Autodesk Inventor part; units mm, degrees
(part 16 of 18)
  line L724 (-5.504, -21.7643) -> (-5.5203, -21.8411)
  arc A19 (7.2375, -23.8979) -> (7.3559, -23.8917) centre (7.2339, -22.6979) ccw
  line L725 (7.7084, -21.9119) -> (7.7586, -22.8684)
  line L726 (6.7189, -22.7122) -> (6.7222, -22.7735)
  arc A20 (9.7799, -23.0242) -> (10.2699, -22.9899) centre (9.9431, -21.8353) ccw
  line L727 (11.0395, -10.3654) -> (11.03, -10.5528)
  line L728 (10.9782, -11.575) -> (10.9727, -11.6853)
  line L729 (10.6615, -17.8311) -> (10.5427, -20.1764)
  line L730 (10.4882, -21.2523) -> (10.4537, -21.9338)
  line L731 (-9.1815, -10.4211) -> (-9.1812, -10.4622)
  line L732 (-9.1335, -17.7807) -> (-9.1304, -18.2698)
  line L733 (8.997, -17.6632) -> (9.1469, -19.1987)
  line L734 (-8.9887, -17.6618) -> (-9.1388, -19.1973)
  line L735 (9.1909, -10.4225) -> (9.1906, -10.4636)
  line L736 (9.1419, -17.7714) -> (9.1385, -18.2712)
  ellipse E590 centre (-10.1862, -4.6596) end of major axis (-11.8856, -4.7023) minor radius 0.2846 (-11.3721, -4.4846) -> (-11.8856, -4.7023) ccw
  line L737 (-11.8818, -4.8559) -> (-11.8856, -4.7023)
  ellipse E591 centre (10.1964, -4.6611) end of major axis (11.8959, -4.7041) minor radius 0.2846 (11.8959, -4.7041) -> (11.3824, -4.4863) ccw
  line L738 (11.892, -4.8577) -> (11.8959, -4.7041)
  ellipse E592 centre (-10.7093, -6.5045) end of major axis (-12.4071, -6.5902) minor radius 0.3038 (-11.6572, -6.2984) -> (-12.4071, -6.5902) ccw
  line L739 (-12.3999, -6.7335) -> (-12.4071, -6.5902)
  ellipse E593 centre (10.7192, -6.5061) end of major axis (12.4171, -6.5921) minor radius 0.3038 (12.4171, -6.5921) -> (11.6673, -6.3002) ccw
  line L740 (12.4098, -6.7354) -> (12.4171, -6.5921)
  ellipse E594 centre (7.1057, -3.5892) end of major axis (8.7977, -3.4241) minor radius 0.0977 (8.7977, -3.4241) -> (8.2803, -3.4043) ccw
  line L741 (8.8221, -3.6736) -> (8.7977, -3.4241)
  ellipse E595 centre (-7.0953, -3.5881) end of major axis (-8.7872, -3.4227) minor radius 0.0977 (-8.2699, -3.403) -> (-8.7872, -3.4227) ccw
  line L742 (-8.8116, -3.6723) -> (-8.7872, -3.4227)
  ellipse E596 centre (-10.1094, -7.7149) end of major axis (-8.6099, -7.6772) minor radius 0.2511 (-9.2363, -7.4893) -> (-9.8598, -7.4611) ccw
  ellipse E597 centre (-10.1094, -7.7149) end of major axis (-8.21, -7.6671) minor radius 0.3181 (-9.2281, -7.4115) -> (-11.1736, -7.4773) ccw
  ellipse E598 centre (-10.1787, -4.9552) end of major axis (-12.0781, -5.003) minor radius 0.3181 (-10.8806, -4.6767) -> (-12.0781, -5.003) ccw
  line L743 (-12.0435, -6.3816) -> (-12.0781, -5.003)
  ellipse E599 centre (7.4558, -8.6381) end of major axis (9.3455, -8.4403) minor radius 0.0812 (9.1873, -8.4899) -> (9.1288, -8.4254) ccw
  ellipse E600 centre (7.1646, -5.8558) end of major axis (9.0543, -5.6581) minor radius 0.0812 (8.9436, -5.6425) -> (8.5431, -5.656) ccw
  line L744 (9.3455, -8.4403) -> (9.1404, -6.481)
  ellipse E601 centre (-7.4461, -8.6369) end of major axis (-9.3358, -8.4389) minor radius 0.0812 (-9.1191, -8.424) -> (-9.1776, -8.4885) ccw
  ellipse E602 centre (-7.1546, -5.8547) end of major axis (-9.0442, -5.6567) minor radius 0.0812 (-8.533, -5.6547) -> (-8.9335, -5.6411) ccw
  line L745 (-9.3358, -8.4389) -> (-9.1305, -6.4796)
  ellipse E603 centre (10.1192, -7.7164) end of major axis (11.6187, -7.7543) minor radius 0.2511 (9.8697, -7.4626) -> (9.2461, -7.4907) ccw
  ellipse E604 centre (10.1192, -7.7164) end of major axis (12.0186, -7.7644) minor radius 0.3181 (11.1834, -7.479) -> (9.238, -7.4129) ccw
  ellipse E605 centre (10.1889, -4.9568) end of major axis (12.0883, -5.0048) minor radius 0.3181 (12.0883, -5.0048) -> (10.8909, -4.6784) ccw
  line L746 (12.0535, -6.3834) -> (12.0883, -5.0048)
  ellipse E606 centre (-10.5555, -9.5507) end of major axis (-12.0536, -9.6263) minor radius 0.2681 (-9.2747, -9.3489) -> (-11.7458, -9.7719) ccw
  ellipse E607 centre (-10.5555, -9.5507) end of major axis (-12.4531, -9.6465) minor radius 0.3396 (-9.2623, -9.2387) -> (-11.7407, -9.8742) ccw
  ellipse E608 centre (-10.6944, -6.7993) end of major axis (-12.592, -6.8951) minor radius 0.3396 (-11.2097, -6.4972) -> (-12.592, -6.8951) ccw
  line L747 (-12.4531, -9.6465) -> (-12.592, -6.8951)
  ellipse E609 centre (7.5123, -10.5929) end of major axis (9.4003, -10.3801) minor radius 0.0405 (9.1011, -10.4359) -> (9.096, -10.3923) ccw
  ellipse E610 centre (7.1988, -7.8111) end of major axis (9.0868, -7.5984) minor radius 0.0405 (9.0374, -7.5948) -> (8.7713, -7.6115) ccw
  line L748 (9.4003, -10.3801) -> (9.1815, -8.4386)
  ellipse E611 centre (-7.5029, -10.5918) end of major axis (-9.3909, -10.3787) minor radius 0.0405 (-9.0866, -10.3909) -> (-9.0917, -10.4345) ccw
  ellipse E612 centre (-7.189, -7.8101) end of major axis (-9.077, -7.597) minor radius 0.0405 (-8.7615, -7.6101) -> (-9.0276, -7.5934) ccw
  line L749 (-9.3909, -10.3787) -> (-9.1718, -8.4372)
  ellipse E613 centre (10.565, -9.5523) end of major axis (12.0631, -9.6282) minor radius 0.2681 (11.7553, -9.7736) -> (9.2843, -9.3503) ccw
  ellipse E614 centre (10.565, -9.5523) end of major axis (12.4626, -9.6484) minor radius 0.3396 (11.7501, -9.8759) -> (9.2718, -9.2401) ccw
  ellipse E615 centre (10.7043, -6.8009) end of major axis (12.6019, -6.897) minor radius 0.3396 (12.6019, -6.897) -> (11.2197, -6.499) ccw
  line L750 (12.4626, -9.6484) -> (12.6019, -6.897)
  ellipse E616 centre (-9.7263, -5.8407) end of major axis (-8.2264, -5.8309) minor radius 0.2359 (-9.2027, -5.6163) -> (-9.2198, -5.6155) ccw
  ellipse E617 centre (-9.7263, -5.8407) end of major axis (-7.8264, -5.8283) minor radius 0.2988 (-9.1962, -5.5504) -> (-10.8665, -5.6089) ccw
  ellipse E618 centre (-9.7443, -3.0756) end of major axis (-11.6443, -3.088) minor radius 0.2988 (-11.5643, -3.0014) -> (-11.6443, -3.088) ccw
  line L751 (-11.6348, -4.5461) -> (-11.6443, -3.088)
  ellipse E619 centre (7.4064, -6.6695) end of major axis (9.2974, -6.4849) minor radius 0.1092 (9.1469, -6.543) -> (9.0264, -6.4553) ccw
  ellipse E620 centre (7.1348, -3.8873) end of major axis (9.0258, -3.7027) minor radius 0.1092 (9.0258, -3.7027) -> (8.3133, -3.6868) ccw
  line L752 (9.2974, -6.4849) -> (9.0258, -3.7027)
  ellipse E621 centre (-7.3965, -6.6683) end of major axis (-9.2874, -6.4835) minor radius 0.1092 (-9.0164, -6.4539) -> (-9.137, -6.5416) ccw
  ellipse E622 centre (-7.1245, -3.8862) end of major axis (-9.0154, -3.7014) minor radius 0.1092 (-8.3029, -3.6856) -> (-9.0154, -3.7014) ccw
  line L753 (-9.2874, -6.4835) -> (-9.0154, -3.7014)
  ellipse E623 centre (9.7364, -5.8422) end of major axis (11.2364, -5.8522) minor radius 0.2359 (9.23, -5.6169) -> (9.2128, -5.6177) ccw
  ellipse E624 centre (9.7364, -5.8422) end of major axis (11.6364, -5.8548) minor radius 0.2988 (10.8767, -5.6106) -> (9.2063, -5.5518) ccw
  ellipse E625 centre (9.7548, -3.0771) end of major axis (11.6548, -3.0897) minor radius 0.2988 (11.6548, -3.0897) -> (11.5748, -3.0032) ccw
  line L754 (11.6451, -4.5478) -> (11.6548, -3.0897)
  line L755 (-8.7402, -12.0526) -> (-8.7237, -12.1531)
  line L756 (-8.7073, -12.253) -> (-7.5133, -19.5411)
  line L757 (-3.535, -19.9576) -> (-2.6762, -17.7502)
  line L758 (-3.5351, -19.9577) -> (-3.535, -19.9576)
  line L759 (-8.1616, -6.5272) -> (-8.5418, -10.158)
  line L760 (-8.7397, -12.0478) -> (-8.7402, -12.0526)
  line L761 (-8.1617, -6.5272) -> (-8.2376, -7.2524)
  line L762 (-3.607, -19.9502) -> (-3.5351, -19.9577)
  line L763 (-7.5133, -19.5411) -> (-7.0907, -19.5854)
  line L764 (-5.4323, -19.759) -> (-3.535, -19.9576)
  ellipse E626 centre (-8.1618, -6.5272) end of major axis (-8.2147, -7.0324) minor radius 0.0001 (-8.1617, -6.5272) -> (-8.1373, -6.2939) ccw
  ellipse E627 centre (-8.1618, -6.5272) end of major axis (-8.2676, -7.5377) minor radius 0.0002 (-8.1616, -6.5272) -> (-8.1128, -6.0606) ccw
  ellipse E628 centre (-7.4804, -0.0138) end of major axis (-7.3746, 0.9967) minor radius 0.0002 (-7.4314, 0.4529) -> (-7.3746, 0.9967) ccw
  ellipse E629 centre (-7.4804, -0.0138) end of major axis (-7.4275, 0.4915) minor radius 0.0001 (-7.4559, 0.2195) -> (-7.4275, 0.4915) ccw
  line L765 (-7.3746, 0.9967) -> (-7.0642, 0.9642)
  line L766 (-8.1373, -6.2939) -> (-7.4559, 0.2195)
  line L767 (-8.1128, -6.0606) -> (-7.4314, 0.4529)
  line L768 (-7.3747, 0.9966) -> (-8.3698, 1.1006)
  line L769 (-8.4227, 0.5954) -> (-8.3698, 1.1006)
  line L770 (-8.4227, 0.5954) -> (-7.4276, 0.4914)
  line L771 (-7.3747, 0.9966) -> (-7.4276, 0.4914)
  line L772 (-8.3698, 1.1006) -> (-8.3699, 1.1006)
  line L773 (-7.4276, 0.4914) -> (-7.4275, 0.4915)
  line L774 (-7.3746, 0.9967) -> (-7.3747, 0.9966)
  line L775 (-3.9949, -5.5989) -> (-3.995, -6.2751)
  line L776 (4.0051, -5.5995) -> (4.005, -6.2757)
  line L777 (-3.9949, -5.5989) -> (-3.9949, -5.1443)
  line L778 (4.0051, -5.5995) -> (4.0051, -5.1449)
  line L779 (-3.9949, -5.1443) -> (-3.9949, -4.6721)
  line L780 (4.0051, -4.6727) -> (4.0051, -5.1449)
  line L781 (4.3271, 1.2542) -> (4.0056, 1.36)
  line L782 (4.0055, 0.8547) -> (4.2649, 0.7694)
  line L783 (-3.9944, 1.3606) -> (-4.3159, 1.2549)
  line L784 (-4.2538, 0.7701) -> (-3.9945, 0.8553)
  line L785 (3.543, -19.9582) -> (3.5431, -19.9582)
  line L786 (2.6845, -17.7506) -> (3.543, -19.9582)
  line L787 (7.5213, -19.5423) -> (8.7164, -12.2543)
  line L788 (8.7328, -12.1544) -> (8.7493, -12.054)
  line L789 (8.2475, -7.2537) -> (8.1717, -6.5284)
  line L790 (8.1716, -6.5284) -> (8.5512, -10.1593)
  line L791 (8.7488, -12.0492) -> (8.7493, -12.054)
  line L792 (3.5431, -19.9582) -> (3.6149, -19.9507)
  line L793 (3.543, -19.9582) -> (5.4402, -19.7598)
  line L794 (7.0987, -19.5864) -> (7.5213, -19.5423)
  ellipse E630 centre (8.1718, -6.5285) end of major axis (8.119, -6.0232) minor radius 0.0001 (8.1473, -6.2951) -> (8.1717, -6.5284) ccw
  ellipse E631 centre (8.1718, -6.5285) end of major axis (8.2774, -7.5389) minor radius 0.0002 (8.1228, -6.0618) -> (8.1716, -6.5284) ccw
  ellipse E632 centre (7.4913, -0.0149) end of major axis (7.3857, 0.9956) minor radius 0.0002 (7.3857, 0.9956) -> (7.4424, 0.4517) ccw
  ellipse E633 centre (7.4913, -0.0149) end of major axis (7.4385, 0.4903) minor radius 0.0001 (7.4385, 0.4903) -> (7.4669, 0.2184) ccw
  line L795 (7.0753, 0.9631) -> (7.3857, 0.9956)
  line L796 (8.1473, -6.2951) -> (7.4669, 0.2184)
  line L797 (7.4424, 0.4517) -> (8.1228, -6.0618)
  line L798 (8.3809, 1.0993) -> (7.3858, 0.9955)
  line L799 (7.4387, 0.4903) -> (7.3858, 0.9955)
  line L800 (7.4387, 0.4903) -> (8.4338, 0.5941)
  line L801 (8.4338, 0.5941) -> (8.3809, 1.0993)
  line L802 (8.381, 1.0993) -> (8.3809, 1.0993)
  line L803 (7.3858, 0.9955) -> (7.3857, 0.9956)
  line L804 (7.4385, 0.4903) -> (7.4387, 0.4903)
  line L805 (-2.9778, -18.5255) -> (-1.9962, -22.1194)
  line L806 (2.0038, -22.1197) -> (2.986, -18.5259)
  line L807 (-1.9962, -22.1194) -> (2.0038, -22.1197)
  line L808 (-2.3716, -21.7977) -> (-1.9963, -23.1626)
  line L809 (2.0037, -23.1629) -> (2.3767, -21.8074)
  line L810 (-1.9963, -23.1626) -> (2.0037, -23.1629)
  line L811 (-8.3636, -21.43) -> (-9.5, -13.9273)
  line L812 (-8.3635, -21.43) -> (-8.3636, -21.43)
  line L813 (-9.5, -13.9273) -> (-8.3635, -21.43)
  line L814 (-9.5, -13.9273) -> (-9.5, -13.9273)
  line L815 (-4.3906, -21.8945) -> (-3.607, -19.9501)
  line L816 (-4.3906, -21.8945) -> (-4.3906, -21.8945)
  line L817 (-8.8548, -8.4092) -> (-9.5, -13.9273)
  line L818 (-8.8549, -8.4092) -> (-9.5, -13.9273)
  line L819 (-8.3636, -21.43) -> (-4.3906, -21.8945)
  line L820 (-8.3635, -21.43) -> (-4.3906, -21.8945)
  ellipse E634 centre (-8.8549, -8.4092) end of major axis (-8.9139, -8.9138) minor radius 0 (-8.8549, -8.4092) -> (-8.8277, -8.1762) ccw
  ellipse E635 centre (-8.8549, -8.4092) end of major axis (-8.9729, -9.4183) minor radius 0.0001 (-8.8548, -8.4092) -> (-8.8004, -7.9432) ccw
  ellipse E636 centre (-8.0948, -1.9044) end of major axis (-7.9768, -0.8953) minor radius 0.0001 (-8.0402, -1.4384) -> (-7.9768, -0.8953) ccw
  ellipse E637 centre (-8.0948, -1.9044) end of major axis (-8.0358, -1.3999) minor radius 0 (-8.0675, -1.6714) -> (-8.0358, -1.3999) ccw
  line L821 (-7.9768, -0.8953) -> (-7.5774, -0.942)
  line L822 (-8.8277, -8.1762) -> (-8.0675, -1.6714)
  line L823 (-8.8004, -7.9432) -> (-8.0402, -1.4384)
  line L824 (-7.9769, -0.8953) -> (-8.9705, -0.7793)
  line L825 (-9.0294, -1.2839) -> (-8.9705, -0.7793)
  line L826 (-9.0294, -1.2839) -> (-8.0359, -1.3999)
  line L827 (-7.9769, -0.8953) -> (-8.0359, -1.3999)
  line L828 (-8.9705, -0.7793) -> (-8.9705, -0.7794)
  line L829 (-8.0359, -1.3999) -> (-8.0358, -1.3999)
  line L830 (-7.9768, -0.8953) -> (-7.9769, -0.8953)
  line L831 (-1.9961, -20.2236) -> (-3.9955, -12.9528)
  line L832 (-1.996, -20.1647) -> (-1.9961, -20.2236)
  line L833 (-3.9955, -12.8939) -> (-1.996, -20.1647)
  line L834 (-3.9955, -12.9528) -> (-3.9955, -12.8939)
  line L835 (4.0045, -12.9534) -> (2.0039, -20.2239)
  line L836 (4.0045, -12.8945) -> (4.0045, -12.9534)
  line L837 (2.004, -20.165) -> (4.0045, -12.8945)
  line L838 (2.0039, -20.2239) -> (2.004, -20.165)
  line L839 (-3.9951, -7.3757) -> (-3.9955, -12.8939)
  line L840 (4.0049, -7.3763) -> (4.0045, -12.8945)
  line L841 (-1.9961, -20.2236) -> (2.0039, -20.2239)
  line L842 (-1.996, -20.1647) -> (2.004, -20.165)
  line L843 (-3.9951, -7.3757) -> (-3.995, -6.923)
  line L844 (4.0049, -7.3763) -> (4.005, -6.9236)
  line L845 (-3.995, -6.923) -> (-3.995, -6.2751)
  line L846 (4.005, -6.2757) -> (4.005, -6.9236)
  line L847 (4.218, -0.5689) -> (4.0054, -0.491)
  line L848 (4.0054, -0.9955) -> (4.158, -1.0515)
  line L849 (-3.9946, -0.4904) -> (-4.2071, -0.5682)
  line L850 (-4.1472, -1.0508) -> (-3.9946, -0.9949)
  line L851 (4.3982, -21.8952) -> (4.3983, -21.8952)
  line L852 (3.6149, -19.9507) -> (4.3982, -21.8952)
  line L853 (9.5089, -13.9287) -> (8.3713, -21.4313)
  line L854 (9.5088, -13.9287) -> (9.5089, -13.9287)
  line L855 (8.3712, -21.4313) -> (9.5088, -13.9287)
  line L856 (8.3713, -21.4313) -> (8.3712, -21.4313)
  line L857 (9.5089, -13.9287) -> (8.8646, -8.4105)
  line L858 (8.8645, -8.4105) -> (9.5088, -13.9287)
  line L859 (4.3983, -21.8952) -> (8.3713, -21.4313)
  line L860 (4.3982, -21.8952) -> (8.3712, -21.4313)
  ellipse E638 centre (8.8646, -8.4105) end of major axis (8.8057, -7.906) minor radius 0 (8.8374, -8.1775) -> (8.8646, -8.4105) ccw
  ellipse E639 centre (8.8646, -8.4105) end of major axis (8.9825, -9.4197) minor radius 0.0001 (8.8101, -7.9445) -> (8.8645, -8.4105) ccw
  ellipse E640 centre (8.1055, -1.9056) end of major axis (7.9876, -0.8965) minor radius 0.0001 (7.9876, -0.8965) -> (8.051, -1.4396) ccw
  ellipse E641 centre (8.1055, -1.9056) end of major axis (8.0465, -1.4011) minor radius 0 (8.0465, -1.4011) -> (8.0782, -1.6726) ccw
  line L861 (7.5882, -0.9431) -> (7.9876, -0.8965)
  line L862 (8.8374, -8.1775) -> (8.0782, -1.6726)
  line L863 (8.051, -1.4396) -> (8.8101, -7.9445)
  line L864 (8.9813, -0.7807) -> (7.9877, -0.8965)
  line L865 (8.0466, -1.4011) -> (7.9877, -0.8965)
  line L866 (8.0466, -1.4011) -> (9.0402, -1.2853)
  line L867 (9.0402, -1.2853) -> (8.9813, -0.7807)
  line L868 (8.9814, -0.7807) -> (8.9813, -0.7807)
  line L869 (7.9877, -0.8965) -> (7.9876, -0.8965)
  line L870 (8.0465, -1.4011) -> (8.0466, -1.4011)
  line L871 (-7.5936, -4.6189) -> (-7.7747, -6.5283)
  line L872 (-7.5936, -4.6189) -> (-7.6627, -5.3469)
  ellipse E642 centre (-7.5936, -4.6189) end of major axis (-7.6416, -5.1246) minor radius 0 (-7.5936, -4.6189) -> (-7.5714, -4.3854) ccw
  ellipse E643 centre (-7.5936, -4.6189) end of major axis (-7.6896, -5.6304) minor radius 0.0001 (-7.5936, -4.6189) -> (-7.5493, -4.1518) ccw
  ellipse E644 centre (-6.9754, 1.901) end of major axis (-6.8794, 2.9125) minor radius 0.0001 (-6.931, 2.3681) -> (-6.8794, 2.9125) ccw
  ellipse E645 centre (-6.9754, 1.901) end of major axis (-6.9274, 2.4068) minor radius 0 (-6.9532, 2.1346) -> (-6.9274, 2.4068) ccw
  line L873 (-6.8794, 2.9125) -> (-4.5993, 2.6962)
  line L874 (-7.5714, -4.3854) -> (-6.9532, 2.1346)
  line L875 (-7.5493, -4.1518) -> (-6.931, 2.3681)
  line L876 (-6.8795, 2.9125) -> (-7.8752, 3.0069)
  line L877 (-7.9232, 2.5012) -> (-7.8752, 3.0069)
  line L878 (-7.9232, 2.5012) -> (-6.9275, 2.4068)
  line L879 (-6.8795, 2.9125) -> (-6.9275, 2.4068)
  line L880 (-7.8752, 3.0069) -> (-7.8754, 3.0069)
  line L881 (-6.9275, 2.4068) -> (-6.9274, 2.4068)
  line L882 (-6.8794, 2.9125) -> (-6.8795, 2.9125)
  line L883 (-3.9948, -3.7775) -> (-3.9949, -4.6721)
  line L884 (4.0052, -3.7782) -> (4.0051, -4.6727)
  line L885 (-3.9948, -3.7775) -> (-3.9948, -3.3213)
  line L886 (4.0052, -3.7782) -> (4.0052, -3.3219)
  line L887 (4.0057, 2.8765) -> (4.0057, 3.3404)
  line L888 (-3.9943, 3.3411) -> (-3.9943, 2.8771)
  line L889 (-3.9943, 3.3411) -> (4.0057, 3.3404)
  line L890 (-3.9948, -3.3213) -> (-3.9943, 2.8771)
  line L891 (4.0057, 2.8765) -> (4.0052, -3.3219)
  line L892 (5.0057, 2.9434) -> (4.0057, 3.2416)
  line L893 (4.0057, 2.7359) -> (4.4825, 2.5937)
  line L894 (5.0057, 2.7329) -> (5.0057, 2.9434)
  line L895 (-3.9943, 3.2422) -> (-4.9943, 2.9442)
  line L896 (-4.9943, 2.7337) -> (-4.9943, 2.9442)
  line L897 (-4.4711, 2.5944) -> (-3.9943, 2.7365)
  line L898 (7.6728, -5.3481) -> (7.6039, -4.62)
  line L899 (7.6038, -4.62) -> (7.7847, -6.5295)
  ellipse E646 centre (7.6039, -4.62) end of major axis (7.556, -4.1143) minor radius 0 (7.5817, -4.3865) -> (7.6039, -4.62) ccw
  ellipse E647 centre (7.6039, -4.62) end of major axis (7.6997, -5.6315) minor radius 0.0001 (7.5596, -4.153) -> (7.6038, -4.62) ccw
  ellipse E648 centre (6.9866, 1.9) end of major axis (6.8908, 2.9115) minor radius 0.0001 (6.8908, 2.9115) -> (6.9423, 2.367) ccw
  ellipse E649 centre (6.9866, 1.9) end of major axis (6.9387, 2.4057) minor radius 0 (6.9387, 2.4057) -> (6.9645, 2.1335) ccw
  line L900 (4.6106, 2.6955) -> (6.8908, 2.9115)
  line L901 (7.5817, -4.3865) -> (6.9645, 2.1335)
  line L902 (6.9423, 2.367) -> (7.5596, -4.153)
  line L903 (7.8867, 3.0057) -> (6.8909, 2.9115)
  line L904 (6.9388, 2.4057) -> (6.8909, 2.9115)
  line L905 (6.9388, 2.4057) -> (7.9346, 2.5)
  line L906 (7.9346, 2.5) -> (7.8867, 3.0057)
  line L907 (7.8868, 3.0057) -> (7.8867, 3.0057)
  line L908 (6.8909, 2.9115) -> (6.8908, 2.9115)
  line L909 (6.9387, 2.4057) -> (6.9388, 2.4057)
  line L910 (-7.7768, -8.2773) -> (-7.756, -8.0785)
  line L911 (-7.7557, -8.0785) -> (-7.7766, -8.2774)
  line L912 (-7.756, -8.0785) -> (-7.7557, -8.0785)
  line L913 (-8.0252, -8.2513) -> (-8.0254, -8.2514)
  line L914 (-7.7766, -8.2774) -> (-8.0252, -8.2513)
  line L915 (-6.782, -8.3815) -> (-6.7612, -8.1826)
  line L916 (-6.5334, -8.4075) -> (-6.782, -8.3815)
  line L917 (-6.7315, -10.2973) -> (-6.9799, -10.2713)
  line L918 (-6.7312, -10.2972) -> (-6.7315, -10.2973)
  line L919 (-7.0007, -10.4701) -> (-6.9799, -10.2712)
  line L920 (-6.9799, -10.2712) -> (-6.7312, -10.2972)
  line L921 (-7.0009, -10.4702) -> (-7.0007, -10.4701)
  line L922 (-7.0009, -10.4702) -> (-7.2651, -10.4425)
  line L923 (-8.2081, -9.9956) -> (-8.0254, -8.2514)
  line L924 (-7.7557, -8.0785) -> (-6.7612, -8.1826)
  line L925 (-6.5334, -8.4075) -> (-6.7312, -10.2972)
  line L926 (-8.2231, -10.141) -> (-8.0252, -8.2513)
  line L927 (-7.0007, -10.4701) -> (-7.9953, -10.3659)
  line L928 (-8.2231, -10.141) -> (-7.9744, -10.167)
  line L929 (-7.9744, -10.167) -> (-7.9953, -10.3659)
  line L930 (-6.8028, -8.5804) -> (-6.959, -10.0723)
  line L931 (-6.959, -10.0723) -> (-7.9536, -9.9681)
  line L932 (-7.9536, -9.9681) -> (-7.7974, -8.4763)
  line L933 (-7.7974, -8.4763) -> (-6.8028, -8.5804)
  line L934 (-7.1162, -9.8786) -> (-6.9967, -8.7375)
  line L935 (-6.959, -10.0723) -> (-7.1162, -9.8786)
  line L936 (-6.8028, -8.5804) -> (-6.9967, -8.7375)
  line L937 (-6.9967, -8.7375) -> (-7.6406, -8.6701)
  line L938 (-7.7974, -8.4763) -> (-7.6406, -8.6701)
  line L939 (-7.6406, -8.6701) -> (-7.76, -9.8112)
  line L940 (-7.9536, -9.9681) -> (-7.76, -9.8112)
  line L941 (-7.76, -9.8112) -> (-7.1162, -9.8786)
  circle A21 centre (-7.3511, -9.0138) radius 0.1
  line L942 (-7.5171, -9.1592) -> (-7.4834, -8.8372)
  line L943 (-7.4834, -8.8372) -> (-7.4834, -8.8372)
  line L944 (-7.5172, -9.1592) -> (-7.4834, -8.8372)
  line L945 (-7.5172, -9.1592) -> (-7.5171, -9.1592)
  line L946 (-7.4834, -8.8372) -> (-7.185, -8.8684)
  line L947 (-7.185, -8.8684) -> (-7.2188, -9.1905)
  line L948 (-7.2188, -9.1905) -> (-7.2188, -9.1905)
  line L949 (-7.2188, -9.1905) -> (-7.5171, -9.1592)
  line L950 (-7.2188, -9.1905) -> (-7.5172, -9.1592)
  line L951 (-6.3909, -18.9045) -> (-6.5898, -18.8837)
  line L952 (-6.3907, -18.9045) -> (-6.3909, -18.9045)
  line L953 (-6.5896, -18.8836) -> (-6.3907, -18.9045)
  line L954 (-6.5898, -18.8837) -> (-6.5896, -18.8836)
  line L955 (-6.4169, -19.1532) -> (-6.3909, -18.9045)
  line L956 (-6.4167, -19.1531) -> (-6.4169, -19.1532)
  line L957 (-6.3907, -18.9045) -> (-6.4167, -19.1531)
  line L958 (-6.2868, -17.9099) -> (-6.2607, -17.6613)
  line L959 (-6.4855, -17.8891) -> (-6.4857, -17.8891)
  line L960 (-6.2865, -17.9099) -> (-6.4855, -17.8891)
  line L961 (-6.2605, -17.6613) -> (-6.2865, -17.9099)
  line L962 (-6.2607, -17.6613) -> (-6.2605, -17.6613)
  line L963 (-6.5898, -18.8837) -> (-6.4857, -17.8891)
  line L964 (-4.5273, -19.351) -> (-6.4169, -19.1532)
  line L965 (-6.5896, -18.8836) -> (-6.4855, -17.8891)
  line L966 (-6.2605, -17.6613) -> (-4.3708, -17.8591)
  line L967 (-4.527, -19.351) -> (-6.4167, -19.1531)
  line L968 (-4.198, -18.1286) -> (-4.3021, -19.1231)
  line L969 (-4.3023, -19.1232) -> (-4.501, -19.1024)
  line L970 (-4.527, -19.351) -> (-4.501, -19.1023)
  line L971 (-4.501, -19.1023) -> (-4.3021, -19.1231)
  line L972 (-4.3021, -19.1231) -> (-4.3023, -19.1232)
  line L973 (-4.5273, -19.351) -> (-4.527, -19.351)
  line L974 (-4.198, -18.1286) -> (-4.3969, -18.1077)
  line L975 (-4.3969, -18.1077) -> (-4.3708, -17.8591)
  line L976 (-6.0876, -17.9307) -> (-4.5958, -18.0869)
  line L977 (-4.5958, -18.0869) -> (-4.6999, -19.0815)
  line L978 (-4.6999, -19.0815) -> (-6.1918, -18.9253)
  line L979 (-6.1918, -18.9253) -> (-6.0876, -17.9307)
  line L980 (-4.7897, -18.244) -> (-5.9308, -18.1245)
  line L981 (-4.5958, -18.0869) -> (-4.7897, -18.244)
  line L982 (-6.0876, -17.9307) -> (-5.9308, -18.1245)
  line L983 (-5.9308, -18.1245) -> (-5.9982, -18.7683)
  line L984 (-6.1918, -18.9253) -> (-5.9982, -18.7683)
  line L985 (-5.9982, -18.7683) -> (-4.8571, -18.8878)
  line L986 (-4.6999, -19.0815) -> (-4.8571, -18.8878)
  line L987 (-4.8571, -18.8878) -> (-4.7897, -18.244)
  circle A22 centre (-5.6544, -18.4789) radius 0.1
  line L988 (-5.509, -18.6449) -> (-5.831, -18.6112)
  line L989 (-5.8311, -18.6112) -> (-5.831, -18.6112)
  line L990 (-5.509, -18.6449) -> (-5.8311, -18.6112)
  line L991 (-5.509, -18.6449) -> (-5.509, -18.6449)
  line L992 (-5.831, -18.6112) -> (-5.7998, -18.3128)
  line L993 (-5.7998, -18.3128) -> (-5.7998, -18.3128)
  line L994 (-5.8311, -18.6112) -> (-5.7998, -18.3128)
  line L995 (-5.7998, -18.3128) -> (-5.4777, -18.3465)
  line L996 (-5.4777, -18.3465) -> (-5.509, -18.6449)
  line L997 (-3.43, -6.9458) -> (-3.4301, -7.1447)
  line L998 (-3.4301, -7.1447) -> (-3.6801, -7.1447)
  line L999 (-2.4301, -7.1448) -> (-2.43, -6.9459)
  line L1000 (-2.1801, -7.1448) -> (-2.4301, -7.1448)
  line L1001 (-3.43, -6.9458) -> (-2.43, -6.9459)
  line L1002 (-2.1801, -7.1448) -> (-2.1802, -8.9028)
  line L1003 (-3.6802, -8.9027) -> (-3.6801, -7.1447)
  line L1004 (-2.4301, -7.3437) -> (-2.4302, -8.7041)
  line L1005 (-3.4302, -8.704) -> (-3.4301, -7.3436)
  line L1006 (-3.4301, -7.3436) -> (-2.4301, -7.3437)
  line L1007 (-2.4301, -7.3437) -> (-2.5901, -7.5972)
  line L1008 (-3.4301, -7.3436) -> (-3.2701, -7.5972)
  ellipse E650 centre (-2.9301, -7.9072) end of major axis (-2.8301, -7.9072) minor radius 0.0995
  ellipse E651 centre (-2.9301, -7.9124) end of major axis (-2.8301, -7.9124) minor radius 0.0995 (-3.0301, -7.9124) -> (-2.8301, -7.9124) ccw
  line L1009 (-3.0301, -7.9124) -> (-3.0301, -7.9072)
  line L1010 (-2.8301, -7.9124) -> (-2.8301, -7.9072)
  line L1011 (-3.0801, -8.0734) -> (-3.0801, -7.7513)
  line L1012 (-3.0801, -8.0839) -> (-3.0801, -8.0734)
  line L1013 (-3.0801, -7.7513) -> (-2.7801, -7.7514)
  line L1014 (-2.7801, -7.7514) -> (-2.7801, -8.0734)
  line L1015 (-2.7801, -8.084) -> (-2.7801, -8.0734)
  line L1016 (-2.7801, -8.0734) -> (-3.0801, -8.0734)
  line L1017 (-1.1458, -17.5133) -> (-0.9458, -17.5133)
  line L1018 (-1.1459, -17.5952) -> (-1.1458, -17.5133)
  line L1019 (-0.9459, -17.762) -> (-0.9459, -17.8436)
  line L1020 (-0.9458, -17.5133) -> (-0.9459, -17.762)
  line L1021 (-0.9458, -16.5187) -> (-1.1458, -16.5187)
  line L1022 (-0.9458, -16.2701) -> (-0.9458, -16.5187)
  line L1023 (-1.1458, -17.5133) -> (-1.1458, -16.5187)
  line L1024 (-0.9458, -16.2701) -> (0.9542, -16.2702)
  line L1025 (0.9541, -17.7621) -> (-0.9459, -17.762)
  line L1026 (1.1542, -16.5189) -> (1.1542, -17.5135)
  line L1027 (0.9541, -17.7621) -> (0.9542, -17.5135)
  line L1028 (0.9542, -17.5135) -> (1.1542, -17.5135)
  line L1029 (1.1542, -17.5135) -> (1.1541, -17.5954)
  line L1030 (0.9541, -17.8437) -> (0.9541, -17.7621)
  line L1031 (1.1542, -16.5189) -> (0.9542, -16.5189)
  line L1032 (0.9542, -16.5189) -> (0.9542, -16.2702)
  line L1033 (-0.7458, -16.5188) -> (0.7542, -16.5189)
  line L1034 (0.7542, -16.5189) -> (0.7542, -17.5134)
  line L1035 (0.7542, -17.5134) -> (-0.7458, -17.5133)
  line L1036 (-0.7458, -17.5133) -> (-0.7458, -16.5188)
  line L1037 (0.7542, -16.5189) -> (0.6136, -16.7417)
  line L1038 (-0.7458, -16.5188) -> (-0.6052, -16.7416)
  line L1039 (-0.7458, -17.5133) -> (-0.6067, -17.4571)
  line L1040 (0.7542, -17.5134) -> (0.6151, -17.4572)
  ellipse E652 centre (-0.2577, -17.0941) end of major axis (-0.1577, -17.0941) minor radius 0.0995
  line L1041 (-0.3577, -17.0986) -> (-0.3577, -17.0941)
  line L1042 (-0.1577, -17.0986) -> (-0.1577, -17.0941)
  line L1043 (4.5091, -19.1031) -> (4.3104, -19.1239)
  line L1044 (4.3102, -19.1238) -> (4.5091, -19.103)
  line L1045 (4.3104, -19.1239) -> (4.3102, -19.1238)
  line L1046 (4.5351, -19.3516) -> (4.5353, -19.3517)
  line L1047 (4.5091, -19.103) -> (4.5351, -19.3516)
  line L1048 (4.4051, -18.1084) -> (4.2062, -18.1292)
  line L1049 (4.3791, -17.8598) -> (4.4051, -18.1084)
  line L1050 (6.269, -17.6623) -> (6.295, -17.9108)
  line L1051 (6.2688, -17.6622) -> (6.269, -17.6623)
  line L1052 (6.4937, -17.8901) -> (6.2948, -17.9109)
  line L1053 (6.2948, -17.9109) -> (6.2688, -17.6622)
  line L1054 (6.4939, -17.8901) -> (6.4937, -17.8901)
  line L1055 (6.4939, -17.8901) -> (6.5979, -18.8847)
  line L1056 (6.425, -19.1542) -> (4.5353, -19.3517)
  line L1057 (4.3102, -19.1238) -> (4.2062, -18.1292)
  line L1058 (4.3791, -17.8598) -> (6.2688, -17.6622)
  line L1059 (6.4248, -19.1541) -> (4.5351, -19.3516)
  line L1060 (6.4937, -17.8901) -> (6.5977, -18.8846)
  line L1061 (6.5979, -18.8847) -> (6.399, -18.9055)
  line L1062 (6.399, -18.9055) -> (6.425, -19.1542)
  line L1063 (6.4248, -19.1541) -> (6.3988, -18.9054)
  line L1064 (6.3988, -18.9054) -> (6.5977, -18.8846)
  line L1065 (6.5977, -18.8846) -> (6.5979, -18.8847)
  line L1066 (6.3988, -18.9054) -> (6.399, -18.9055)
  line L1067 (6.425, -19.1542) -> (6.4248, -19.1541)
  line L1068 (4.604, -18.0876) -> (6.0959, -17.9316)
  line L1069 (6.0959, -17.9316) -> (6.1999, -18.9262)
  line L1070 (6.1999, -18.9262) -> (4.708, -19.0822)
  line L1071 (4.708, -19.0822) -> (4.604, -18.0876)
  line L1072 (5.939, -18.1254) -> (4.7979, -18.2447)
  line L1073 (6.0959, -17.9316) -> (5.939, -18.1254)
  line L1074 (4.604, -18.0876) -> (4.7979, -18.2447)
  line L1075 (4.7979, -18.2447) -> (4.8652, -18.8885)
  line L1076 (4.708, -19.0822) -> (4.8652, -18.8885)
  line L1077 (4.8652, -18.8885) -> (6.0063, -18.7692)
  line L1078 (6.1999, -18.9262) -> (6.0063, -18.7692)
  line L1079 (6.0063, -18.7692) -> (5.939, -18.1254)
  circle A23 centre (5.1416, -18.5342) radius 0.1
  line L1080 (5.3182, -18.6666) -> (4.9961, -18.7002)
  line L1081 (4.9962, -18.7002) -> (4.9961, -18.7002)
  line L1082 (5.3182, -18.6666) -> (4.9962, -18.7002)
  line L1083 (5.3182, -18.6666) -> (5.3182, -18.6666)
  line L1084 (4.9961, -18.7002) -> (4.9649, -18.4019)
  line L1085 (4.9649, -18.4019) -> (5.287, -18.3682)
  line L1086 (5.287, -18.3682) -> (5.287, -18.3682)
  line L1087 (5.287, -18.3682) -> (5.3182, -18.6666)
  line L1088 (5.287, -18.3682) -> (5.3182, -18.6666)
  line L1089 (-1.1461, -21.3694) -> (-0.9461, -21.3694)
  line L1090 (-0.9461, -21.3694) -> (-0.9462, -21.6194)
  line L1091 (-0.9461, -20.3694) -> (-1.1461, -20.3694)
  line L1092 (-0.9461, -20.2237) -> (-0.9461, -20.3694)
  line L1093 (-1.1461, -21.3694) -> (-1.1461, -20.3694)
  line L1094 (0.9538, -21.6196) -> (-0.9462, -21.6194)
  line L1095 (1.1539, -20.3696) -> (1.1539, -21.3696)
  line L1096 (0.9538, -21.6196) -> (0.9539, -21.3696)
  line L1097 (0.9539, -21.3696) -> (1.1539, -21.3696)
  line L1098 (1.1539, -20.3696) -> (0.9539, -20.3696)
  line L1099 (0.9539, -20.3696) -> (0.9539, -20.2239)
  line L1100 (-0.7461, -20.3694) -> (0.7539, -20.3696)
  line L1101 (0.7539, -20.3696) -> (0.7539, -21.3696)
  line L1102 (0.7539, -21.3696) -> (-0.7461, -21.3694)
  line L1103 (-0.7461, -21.3694) -> (-0.7461, -20.3694)
  line L1104 (0.5776, -20.5459) -> (-0.5698, -20.5458)
  line L1105 (0.7539, -20.3696) -> (0.5776, -20.5459)
  line L1106 (-0.7461, -20.3694) -> (-0.5698, -20.5458)
  line L1107 (-0.5698, -20.5458) -> (-0.5698, -21.1931)
  line L1108 (-0.7461, -21.3694) -> (-0.5698, -21.1931)
  line L1109 (-0.5698, -21.1931) -> (0.5775, -21.1932)
  line L1110 (0.7539, -21.3696) -> (0.5775, -21.1932)
  line L1111 (0.5775, -21.1932) -> (0.5776, -20.5459)
  circle A24 centre (-0.258, -20.8695) radius 0.1
  line L1112 (-0.0961, -21.0195) -> (-0.4199, -21.0195)
  line L1113 (-0.4199, -21.0195) -> (-0.4199, -20.7195)
  line L1114 (-0.4199, -20.7195) -> (-0.0961, -20.7195)
  line L1115 (-0.0961, -20.7195) -> (-0.0961, -21.0195)
  line L1116 (-1.1462, -22.5801) -> (-0.9462, -22.5801)
  line L1117 (-0.9462, -22.5801) -> (-0.9463, -22.8284)
  line L1118 (-1.1462, -22.5801) -> (-1.1462, -22.1194)
  line L1119 (0.9537, -22.8286) -> (-0.9463, -22.8284)
  line L1120 (1.1538, -22.1196) -> (1.1538, -22.5803)
  line L1121 (0.9537, -22.8286) -> (0.9538, -22.5802)
  line L1122 (0.9538, -22.5802) -> (1.1538, -22.5803)
  line L1123 (0.7538, -22.1196) -> (0.7538, -22.5802)
  line L1124 (0.7538, -22.5802) -> (-0.7462, -22.5801)
  line L1125 (-0.7462, -22.5801) -> (-0.7462, -22.1194)
  line L1126 (-0.5699, -22.1195) -> (-0.5699, -22.289)
  line L1127 (-0.7462, -22.5801) -> (-0.5699, -22.289)
  line L1128 (-0.5699, -22.289) -> (0.5775, -22.2891)
  line L1129 (0.7538, -22.5802) -> (0.5775, -22.2891)
  line L1130 (0.5775, -22.2891) -> (0.5775, -22.1195)
  line L1131 (-0.0962, -22.1397) -> (-0.42, -22.1397)
  line L1132 (-0.42, -22.1397) -> (-0.42, -22.1195)
  line L1133 (-0.0962, -22.1195) -> (-0.0962, -22.1397)
  line L1134 (-8.4678, -9.9653) -> (-8.491, -10.1639)
  line L1135 (-8.4679, -9.9653) -> (-8.4678, -9.9653)
  line L1136 (-8.7393, -10.1349) -> (-8.7395, -10.1349)
  line L1137 (-8.491, -10.1639) -> (-8.7393, -10.1349)
  line L1138 (-8.7073, -12.253) -> (-8.735, -12.2498)
  line L1139 (-8.9601, -12.0221) -> (-8.7395, -10.1349)
  line L1140 (-8.4678, -9.9653) -> (-8.2079, -9.9956)
  line L1141 (-7.2651, -10.4424) -> (-7.4701, -12.1962)
  line L1142 (-8.96, -12.022) -> (-8.7393, -10.1349)
  line L1143 (-7.7416, -12.3658) -> (-8.7349, -12.2497)
  line L1144 (-8.735, -12.2498) -> (-8.7237, -12.1531)
  line L1145 (-8.7397, -12.0478) -> (-8.9601, -12.0221)
  line L1146 (-8.96, -12.022) -> (-8.7116, -12.051)
  line L1147 (-8.7116, -12.051) -> (-8.7349, -12.2497)
  line L1148 (-8.7349, -12.2497) -> (-8.735, -12.2498)
  line L1149 (-8.7116, -12.051) -> (-8.7118, -12.0511)
  line L1150 (-8.9601, -12.0221) -> (-8.96, -12.022)
  line L1151 (-7.4701, -12.1962) -> (-7.4702, -12.1963)
  line L1152 (-7.7416, -12.3658) -> (-7.7184, -12.1672)
  line L1153 (-7.7184, -12.1672) -> (-7.4701, -12.1962)
  line L1154 (-7.7418, -12.3659) -> (-7.7416, -12.3658)
  line L1155 (-7.521, -10.4787) -> (-7.6952, -11.9685)
  line L1156 (-7.6952, -11.9685) -> (-8.6884, -11.8524)
  line L1157 (-8.6884, -11.8524) -> (-8.5142, -10.3625)
  line L1158 (-8.5142, -10.3625) -> (-7.521, -10.4787)
  line L1159 (-7.8499, -11.773) -> (-7.7167, -10.6334)
  line L1160 (-7.6952, -11.9685) -> (-7.8499, -11.773)
  line L1161 (-7.521, -10.4787) -> (-7.7167, -10.6334)
  line L1162 (-7.7167, -10.6334) -> (-8.3597, -10.5582)
  line L1163 (-8.5142, -10.3625) -> (-8.3597, -10.5582)
  line L1164 (-8.3597, -10.5582) -> (-8.4929, -11.6978)
  line L1165 (-8.6884, -11.8524) -> (-8.4929, -11.6978)
  line L1166 (-8.4929, -11.6978) -> (-7.8499, -11.773)
  circle A25 centre (-8.0744, -10.9054) radius 0.1
  line L1167 (-8.2422, -11.0488) -> (-8.2046, -10.7272)
  line L1168 (-8.2046, -10.7272) -> (-8.2046, -10.7272)
  line L1169 (-8.2422, -11.0488) -> (-8.2046, -10.7272)
  line L1170 (-8.2422, -11.0488) -> (-8.2422, -11.0488)
  line L1171 (-8.2046, -10.7272) -> (-7.9066, -10.762)
  line L1172 (-7.9066, -10.762) -> (-7.9442, -11.0837)
  line L1173 (-7.9442, -11.0837) -> (-7.9442, -11.0837)
  line L1174 (-7.9442, -11.0837) -> (-8.2422, -11.0488)
  line L1175 (-7.9442, -11.0837) -> (-8.2422, -11.0488)
  line L1176 (-7.2335, -20.807) -> (-7.4322, -20.7838)
  line L1177 (-7.2334, -20.8069) -> (-7.2335, -20.807)
  line L1178 (-7.4321, -20.7837) -> (-7.2334, -20.8069)
  line L1179 (-7.4322, -20.7838) -> (-7.4321, -20.7837)
  line L1180 (-7.2626, -21.0553) -> (-7.2335, -20.807)
  line L1181 (-7.2624, -21.0553) -> (-7.2626, -21.0553)
  line L1182 (-7.2334, -20.8069) -> (-7.2624, -21.0553)
  line L1183 (-7.1174, -19.8137) -> (-7.0907, -19.5854)
  line L1184 (-7.3159, -19.7905) -> (-7.3161, -19.7905)
  line L1185 (-7.1173, -19.8137) -> (-7.3159, -19.7905)
  line L1186 (-7.0883, -19.5654) -> (-7.1173, -19.8137)
  line L1187 (-7.0884, -19.5655) -> (-7.0883, -19.5654)
  line L1188 (-7.4322, -20.7838) -> (-7.3161, -19.7905)
  line L1189 (-5.3754, -21.2759) -> (-7.2626, -21.0553)
  line L1190 (-7.4321, -20.7837) -> (-7.3159, -19.7905)
  line L1191 (-7.0883, -19.5654) -> (-5.2011, -19.786)
  line L1192 (-5.3753, -21.2759) -> (-7.2624, -21.0553)
  line L1193 (-5.0315, -20.0576) -> (-5.1476, -21.0508)
  line L1194 (-5.1478, -21.0509) -> (-5.3463, -21.0276)
  line L1195 (-5.3753, -21.2759) -> (-5.3463, -21.0276)
  line L1196 (-5.3463, -21.0276) -> (-5.1476, -21.0508)
  line L1197 (-5.1476, -21.0508) -> (-5.1478, -21.0509)
  line L1198 (-5.3754, -21.2759) -> (-5.3753, -21.2759)
  line L1199 (-5.0315, -20.0576) -> (-5.2301, -20.0343)
  line L1200 (-5.2301, -20.0343) -> (-5.2011, -19.786)
  line L1201 (-6.9186, -19.8369) -> (-5.4288, -20.0111)
  line L1202 (-5.4288, -20.0111) -> (-5.5449, -21.0044)
  line L1203 (-5.5449, -21.0044) -> (-7.0348, -20.8302)
  line L1204 (-7.0348, -20.8302) -> (-6.9186, -19.8369)
  line L1205 (-5.6245, -20.1658) -> (-6.7641, -20.0326)
  line L1206 (-5.4288, -20.0111) -> (-5.6245, -20.1658)
  line L1207 (-6.9186, -19.8369) -> (-6.7641, -20.0326)
  line L1208 (-6.7641, -20.0326) -> (-6.8393, -20.6755)
  line L1209 (-7.0348, -20.8302) -> (-6.8393, -20.6755)
  line L1210 (-6.8393, -20.6755) -> (-5.6997, -20.8088)
  line L1211 (-5.5449, -21.0044) -> (-5.6997, -20.8088)
  line L1212 (-5.6997, -20.8088) -> (-5.6245, -20.1658)
  circle A26 centre (-6.492, -20.3903) radius 0.1
  line L1213 (-6.3486, -20.558) -> (-6.6702, -20.5204)
  line L1214 (-6.6702, -20.5204) -> (-6.6702, -20.5204)
  line L1215 (-6.3486, -20.5581) -> (-6.6702, -20.5204)
  line L1216 (-6.3486, -20.5581) -> (-6.3486, -20.558)
  line L1217 (-6.6702, -20.5204) -> (-6.6354, -20.2225)
  line L1218 (-6.6354, -20.2225) -> (-6.6354, -20.2225)
  line L1219 (-6.6702, -20.5204) -> (-6.6354, -20.2225)
  line L1220 (-6.6354, -20.2225) -> (-6.3138, -20.2601)
  line L1221 (-6.3138, -20.2601) -> (-6.3486, -20.558)
  line L1222 (-3.4302, -8.704) -> (-3.4302, -8.9027)
  line L1223 (-3.4302, -8.9027) -> (-3.6802, -8.9027)
  line L1224 (-2.4302, -8.9028) -> (-2.4302, -8.7041)
  line L1225 (-2.1802, -8.9028) -> (-2.4302, -8.9028)
  line L1226 (-2.1803, -10.9523) -> (-2.4303, -10.9522)
  line L1227 (-2.1803, -10.79) -> (-2.1803, -10.9523)
  line L1228 (-2.4304, -10.9886) -> (-2.4303, -10.7899)
  line L1229 (-2.4303, -10.7899) -> (-2.1803, -10.79)
  line L1230 (-2.4304, -11.1509) -> (-2.4304, -10.9886)
  line L1231 (-2.4304, -11.1509) -> (-3.4304, -11.1508)
  line L1232 (-3.4302, -8.704) -> (-2.4302, -8.7041)
  line L1233 (-2.1802, -8.9028) -> (-2.1803, -10.79)
  line L1234 (-3.6803, -10.7899) -> (-3.6802, -8.9027)
  line L1235 (-2.4304, -10.9886) -> (-3.4304, -10.9885)
  line L1236 (-3.4303, -10.9522) -> (-3.6803, -10.9521)
  line L1237 (-3.6803, -10.7899) -> (-3.4303, -10.7899)
  line L1238 (-3.4303, -10.7899) -> (-3.4304, -10.9885)
  line L1239 (-3.4304, -10.9885) -> (-3.4304, -11.1508)
  line L1240 (-3.6803, -10.9521) -> (-3.6803, -10.7899)
  line L1241 (-2.4302, -9.1014) -> (-2.4303, -10.5913)
  line L1242 (-2.4303, -10.5913) -> (-3.4303, -10.5912)
  line L1243 (-3.4303, -10.5912) -> (-3.4302, -9.1013)
  line L1244 (-3.4302, -9.1013) -> (-2.4302, -9.1014)
  line L1245 (-2.6066, -10.5321) -> (-2.6066, -9.3924)
  line L1246 (-2.4303, -10.5913) -> (-2.6066, -10.5321)
  line L1247 (-2.4302, -9.1014) -> (-2.6066, -9.3924)
  line L1248 (-2.6066, -9.3924) -> (-3.2539, -9.3924)
  line L1249 (-3.4302, -9.1013) -> (-3.2539, -9.3924)
  line L1250 (-3.2539, -9.3924) -> (-3.254, -10.532)
  line L1251 (-3.4303, -10.5912) -> (-3.254, -10.532)
  line L1252 (-3.254, -10.532) -> (-2.6066, -10.5321)
  ellipse E653 centre (-2.9303, -9.6731) end of major axis (-2.8303, -9.6731) minor radius 0.0993
  ellipse E654 centre (-2.9303, -9.6789) end of major axis (-2.8303, -9.6789) minor radius 0.0993 (-3.0303, -9.6789) -> (-2.8303, -9.6789) ccw
  line L1253 (-3.0303, -9.6789) -> (-3.0303, -9.6731)
  line L1254 (-2.8303, -9.6789) -> (-2.8303, -9.6731)
  line L1255 (-3.0803, -9.8397) -> (-3.0802, -9.5181)
  line L1256 (-3.0803, -9.8629) -> (-3.0803, -9.8397)
  line L1257 (-3.0802, -9.5181) -> (-2.7802, -9.5181)
  line L1258 (-2.7802, -9.5181) -> (-2.7803, -9.8397)
  line L1259 (-2.7803, -9.8629) -> (-2.7803, -9.8397)
  line L1260 (-2.7803, -9.8397) -> (-3.0803, -9.8397)
  line L1261 (-2.7803, -9.8629) -> (-3.0803, -9.8629)
  line L1262 (-0.946, -19.4199) -> (-1.146, -19.4199)
  line L1263 (-1.146, -19.2576) -> (-0.946, -19.2576)
  line L1264 (-1.146, -19.4199) -> (-1.146, -19.2576)
  line L1265 (-0.946, -19.5059) -> (-0.946, -19.6682)
  line L1266 (-0.946, -19.2576) -> (-0.946, -19.5059)
  line L1267 (-0.9459, -18.2643) -> (-1.1459, -18.2643)
  line L1268 (-0.9459, -18.016) -> (-0.9459, -18.2643)
  line L1269 (1.154, -19.42) -> (0.954, -19.42)
  line L1270 (0.954, -19.506) -> (0.954, -19.2577)
  line L1271 (0.954, -19.2577) -> (1.154, -19.2577)
  line L1272 (1.154, -19.2577) -> (1.154, -19.42)
  line L1273 (0.954, -19.6683) -> (0.954, -19.506)
  line L1274 (0.954, -19.6683) -> (-0.946, -19.6682)
  line L1275 (-1.146, -19.2576) -> (-1.1459, -18.2643)
  line L1276 (-0.9459, -18.016) -> (0.9541, -18.0162)
  line L1277 (0.954, -19.506) -> (-0.946, -19.5059)
  line L1278 (1.1541, -18.2645) -> (1.154, -19.2577)
  line L1279 (1.1541, -18.2645) -> (0.9541, -18.2645)
  line L1280 (0.9541, -18.2645) -> (0.9541, -18.0162)
  line L1281 (-0.7459, -18.2643) -> (0.7541, -18.2645)
  line L1282 (0.7541, -18.2645) -> (0.754, -19.2577)
  line L1283 (0.754, -19.2577) -> (-0.746, -19.2576)
  line L1284 (-0.746, -19.2576) -> (-0.7459, -18.2643)
  line L1285 (0.5777, -18.5555) -> (-0.5696, -18.5554)
  line L1286 (0.7541, -18.2645) -> (0.5777, -18.5555)
  line L1287 (-0.7459, -18.2643) -> (-0.5696, -18.5554)
  line L1288 (-0.5696, -18.5554) -> (-0.5696, -19.1984)
  line L1289 (-0.746, -19.2576) -> (-0.5696, -19.1984)
  line L1290 (-0.5696, -19.1984) -> (0.5777, -19.1985)
  line L1291 (0.754, -19.2577) -> (0.5777, -19.1985)
  line L1292 (0.5777, -19.1985) -> (0.5777, -18.5555)
  ellipse E655 centre (-0.2579, -18.848) end of major axis (-0.1579, -18.848) minor radius 0.0993
  ellipse E656 centre (-0.2579, -18.8537) end of major axis (-0.1579, -18.8538) minor radius 0.0993 (-0.3579, -18.8537) -> (-0.1579, -18.8538) ccw
  line L1293 (-0.3579, -18.8537) -> (-0.3579, -18.8479)
  line L1294 (-0.1579, -18.8538) -> (-0.1579, -18.848)
  line L1295 (-0.096, -19.0027) -> (-0.4198, -19.0027)
  line L1296 (-0.4198, -19.0259) -> (-0.4198, -19.0027)
  line L1297 (-0.096, -19.0259) -> (-0.4198, -19.0259)
  line L1298 (-0.096, -19.0259) -> (-0.096, -19.0027)
  line L1299 (-0.4198, -19.0027) -> (-0.4198, -18.7047)
  line L1300 (-0.4198, -18.7047) -> (-0.0959, -18.7048)
  line L1301 (-0.0959, -18.7048) -> (-0.096, -19.0027)
  line L1302 (5.354, -21.0285) -> (5.1555, -21.0516)
  line L1303 (5.1554, -21.0516) -> (5.354, -21.0284)
  line L1304 (5.1555, -21.0516) -> (5.1554, -21.0516)
  line L1305 (5.383, -21.2767) -> (5.3832, -21.2768)
  line L1306 (5.354, -21.0284) -> (5.383, -21.2767)
  line L1307 (5.2381, -20.0351) -> (5.0394, -20.0583)
  line L1308 (5.2091, -19.7868) -> (5.2381, -20.0351)
  line L1309 (7.0987, -19.5864) -> (7.1254, -19.8148)
  line L1310 (7.0962, -19.5665) -> (7.0964, -19.5665)
  line L1311 (7.3239, -19.7916) -> (7.1252, -19.8148)
  line L1312 (7.1252, -19.8148) -> (7.0962, -19.5665)
  line L1313 (7.324, -19.7917) -> (7.3239, -19.7916)
  line L1314 (7.324, -19.7917) -> (7.44, -20.7849)
  line L1315 (7.2703, -21.0564) -> (5.3832, -21.2768)
  line L1316 (5.1554, -21.0516) -> (5.0394, -20.0583)
  line L1317 (5.2091, -19.7868) -> (7.0962, -19.5665)
  line L1318 (7.2702, -21.0564) -> (5.383, -21.2767)
  line L1319 (7.3239, -19.7916) -> (7.4399, -20.7848)
  line L1320 (7.44, -20.7849) -> (7.2414, -20.8081)
  line L1321 (7.2414, -20.8081) -> (7.2703, -21.0564)
  line L1322 (7.2702, -21.0564) -> (7.2412, -20.808)
  line L1323 (7.2412, -20.808) -> (7.4399, -20.7848)
  line L1324 (7.4399, -20.7848) -> (7.44, -20.7849)
  line L1325 (7.2412, -20.808) -> (7.2414, -20.8081)
  line L1326 (7.2703, -21.0564) -> (7.2702, -21.0564)
  line L1327 (5.4367, -20.0119) -> (6.9266, -19.838)
  line L1328 (6.9266, -19.838) -> (7.0426, -20.8312)
  line L1329 (7.0426, -20.8312) -> (5.5527, -21.0052)
  line L1330 (5.5527, -21.0052) -> (5.4367, -20.0119)
  line L1331 (6.772, -20.0336) -> (5.6324, -20.1667)
  line L1332 (6.9266, -19.838) -> (6.772, -20.0336)
  line L1333 (5.4367, -20.0119) -> (5.6324, -20.1667)
  line L1334 (5.6324, -20.1667) -> (5.7075, -20.8096)
  line L1335 (5.5527, -21.0052) -> (5.7075, -20.8096)
  line L1336 (5.7075, -20.8096) -> (6.8471, -20.6766)
  line L1337 (7.0426, -20.8312) -> (6.8471, -20.6766)
  line L1338 (6.8471, -20.6766) -> (6.772, -20.0336)
  circle A27 centre (5.9796, -20.452) radius 0.1
  line L1339 (6.1578, -20.5822) -> (5.8361, -20.6198)
  line L1340 (5.8362, -20.6198) -> (5.8361, -20.6198)
  line L1341 (6.1578, -20.5822) -> (5.8362, -20.6198)
  line L1342 (6.1578, -20.5822) -> (6.1578, -20.5822)
  line L1343 (5.8361, -20.6198) -> (5.8014, -20.3218)
  line L1344 (5.8014, -20.3218) -> (6.123, -20.2842)
  line L1345 (6.123, -20.2842) -> (6.123, -20.2842)
  line L1346 (6.123, -20.2842) -> (6.1578, -20.5822)
  line L1347 (6.123, -20.2842) -> (6.1578, -20.5822)
  line L1348 (-7.1917, -6.3653) -> (-7.1728, -6.1662)
  line L1349 (-7.1727, -6.1662) -> (-7.1916, -6.3653)
  line L1350 (-7.1728, -6.1662) -> (-7.1727, -6.1662)
  line L1351 (-7.4405, -6.3417) -> (-7.4406, -6.3417)
  line L1352 (-7.1916, -6.3653) -> (-7.4405, -6.3417)
  line L1353 (-6.1961, -6.4598) -> (-6.1772, -6.2607)
  line L1354 (-5.9472, -6.4834) -> (-6.1961, -6.4598)
  line L1355 (-7.4615, -6.5618) -> (-7.4406, -6.3417)
  line L1356 (-7.1727, -6.1662) -> (-6.1772, -6.2607)
  line L1357 (-5.9472, -6.4834) -> (-6.1266, -8.3749)
  line L1358 (-7.6067, -8.0941) -> (-7.4405, -6.3417)
  line L1359 (-6.3944, -8.5504) -> (-6.5468, -8.5359)
  line L1360 (-6.1266, -8.3749) -> (-6.1267, -8.3749)
  line L1361 (-6.3944, -8.5504) -> (-6.3755, -8.3513)
  line L1362 (-6.3755, -8.3513) -> (-6.1266, -8.3749)
  line L1363 (-6.3945, -8.5504) -> (-6.3944, -8.5504)
  line L1364 (-6.2149, -6.6589) -> (-6.3566, -8.1522)
  line L1365 (-6.3566, -8.1522) -> (-7.3521, -8.0577)
  line L1366 (-7.3521, -8.0577) -> (-7.2105, -6.5644)
  line L1367 (-7.2105, -6.5644) -> (-6.2149, -6.6589)
  line L1368 (-6.5156, -7.96) -> (-6.4072, -6.8178)
  line L1369 (-6.3566, -8.1522) -> (-6.5156, -7.96)
  line L1370 (-6.2149, -6.6589) -> (-6.4072, -6.8178)
  line L1371 (-6.4072, -6.8178) -> (-7.0517, -6.7566)
  line L1372 (-7.2105, -6.5644) -> (-7.0517, -6.7566)
  line L1373 (-7.0517, -6.7566) -> (-7.16, -7.8989)
  line L1374 (-7.3521, -8.0577) -> (-7.16, -7.8989)
  line L1375 (-7.16, -7.8989) -> (-6.5156, -7.96)
  circle A28 centre (-6.7589, -7.0976) radius 0.1
  line L1376 (-6.9235, -7.2446) -> (-6.8929, -6.9222)
  line L1377 (-6.9235, -7.2446) -> (-6.8929, -6.9222)
  line L1378 (-6.8929, -6.9222) -> (-6.5942, -6.9505)
  line L1379 (-6.5942, -6.9505) -> (-6.6248, -7.2729)
  line L1380 (-6.6248, -7.2729) -> (-6.9235, -7.2446)
  line L1381 (-5.7022, -16.9784) -> (-5.7023, -16.9784)
  line L1382 (-5.9013, -16.9595) -> (-5.7022, -16.9784)
  line L1383 (-5.9014, -16.9595) -> (-5.9013, -16.9595)
  line L1384 (-5.7258, -17.2273) -> (-5.7259, -17.2273)
  line L1385 (-5.7022, -16.9784) -> (-5.7258, -17.2273)
  line L1386 (-5.8069, -15.964) -> (-5.807, -15.964)
  line L1387 (-5.6078, -15.9829) -> (-5.8069, -15.964)
  line L1388 (-5.5842, -15.734) -> (-5.6078, -15.9829)
  line L1389 (-5.5843, -15.734) -> (-5.5842, -15.734)
  line L1390 (-5.9013, -16.9595) -> (-5.8069, -15.964)
  line L1391 (-5.5842, -15.734) -> (-3.6927, -15.9134)
  line L1392 (-3.8343, -17.4067) -> (-5.7258, -17.2273)
  line L1393 (-3.5172, -16.1812) -> (-3.6116, -17.1767)
  line L1394 (-3.8343, -17.4067) -> (-3.8107, -17.1579)
  line L1395 (-3.8107, -17.1579) -> (-3.6116, -17.1767)
  line L1396 (-3.6116, -17.1767) -> (-3.6117, -17.1767)
  line L1397 (-3.8344, -17.4067) -> (-3.8343, -17.4067)
  line L1398 (-3.5172, -16.1812) -> (-3.7163, -16.1623)
  line L1399 (-3.7163, -16.1623) -> (-3.6927, -15.9134)
  line L1400 (-5.4087, -16.0018) -> (-3.9154, -16.1434)
  line L1401 (-3.9154, -16.1434) -> (-4.0098, -17.139)
  line L1402 (-4.0098, -17.139) -> (-5.5031, -16.9973)
  line L1403 (-5.5031, -16.9973) -> (-5.4087, -16.0018)
  line L1404 (-4.1076, -16.3023) -> (-5.2499, -16.194)
  line L1405 (-3.9154, -16.1434) -> (-4.1076, -16.3023)
  line L1406 (-5.4087, -16.0018) -> (-5.2499, -16.194)
  line L1407 (-5.2499, -16.194) -> (-5.311, -16.8384)
  line L1408 (-5.5031, -16.9973) -> (-5.311, -16.8384)
  line L1409 (-5.311, -16.8384) -> (-4.1688, -16.9468)
  line L1410 (-4.0098, -17.139) -> (-4.1688, -16.9468)
  line L1411 (-4.1688, -16.9468) -> (-4.1076, -16.3023)
  circle A29 centre (-4.97, -16.5456) radius 0.1
  line L1412 (-4.823, -16.7103) -> (-5.1454, -16.6797)
  line L1413 (-5.1454, -16.6797) -> (-5.1171, -16.381)
  line L1414 (-5.1454, -16.6797) -> (-5.1171, -16.381)
  line L1415 (-5.1171, -16.381) -> (-4.7947, -16.4116)
  line L1416 (-4.7947, -16.4116) -> (-4.823, -16.7103)
  line L1417 (-3.4299, -5.1395) -> (-3.4299, -5.3386)
  line L1418 (-3.4299, -5.3386) -> (-3.6799, -5.3386)
  line L1419 (-2.4299, -5.3387) -> (-2.4299, -5.1396)
  line L1420 (-2.1799, -5.3387) -> (-2.4299, -5.3387)
  line L1421 (-3.4299, -5.1395) -> (-2.4299, -5.1396)
  line L1422 (-2.1799, -5.3387) -> (-2.1801, -7.1448)
  line L1423 (-3.6801, -7.1447) -> (-3.6799, -5.3386)
  line L1424 (-2.4299, -5.5378) -> (-2.43, -6.9459)
  line L1425 (-3.43, -6.9458) -> (-3.4299, -5.5378)
  line L1426 (-3.4299, -5.5378) -> (-2.4299, -5.5378)
  line L1427 (-2.6063, -6.2884) -> (-2.6063, -5.8077)
  line L1428 (-2.4299, -5.5378) -> (-2.6063, -5.8077)
  line L1429 (-2.6063, -5.8077) -> (-3.2536, -5.8076)
  line L1430 (-3.4299, -5.5378) -> (-3.2536, -5.8076)
  line L1431 (-3.2536, -5.8076) -> (-3.2537, -6.2883)
  ellipse E657 centre (-2.93, -6.0945) end of major axis (-2.83, -6.0945) minor radius 0.0996
  ellipse E658 centre (-2.93, -6.0992) end of major axis (-2.83, -6.0992) minor radius 0.0996 (-3.03, -6.0992) -> (-2.83, -6.0992) ccw
  line L1432 (-3.03, -6.0992) -> (-3.03, -6.0944)
  line L1433 (-2.83, -6.0992) -> (-2.83, -6.0945)
  line L1434 (-3.08, -6.2603) -> (-3.08, -5.938)
  line L1435 (-3.08, -6.2792) -> (-3.08, -6.2603)
  line L1436 (-3.08, -5.938) -> (-2.78, -5.938)
  line L1437 (-2.78, -5.938) -> (-2.78, -6.2604)
  line L1438 (-2.78, -6.2792) -> (-2.78, -6.2604)
  line L1439 (-2.78, -6.2604) -> (-3.08, -6.2603)
  line L1440 (-2.78, -6.2792) -> (-3.08, -6.2792)
  line L1441 (-1.1457, -15.7173) -> (-0.9457, -15.7174)
  line L1442 (-1.1457, -15.7478) -> (-1.1457, -15.7173)
  line L1443 (-0.9457, -15.9662) -> (-0.9457, -15.9962)
  line L1444 (-0.9457, -15.7174) -> (-0.9457, -15.9662)
  line L1445 (-0.9456, -14.7218) -> (-1.1456, -14.7218)
  line L1446 (-0.9456, -14.4729) -> (-0.9456, -14.7218)
  line L1447 (-1.1457, -15.7173) -> (-1.1456, -14.7218)
  line L1448 (-0.9456, -14.4729) -> (0.9544, -14.4731)
  line L1449 (0.9543, -15.9664) -> (-0.9457, -15.9662)
  line L1450 (1.1544, -14.722) -> (1.1543, -15.7175)
  line L1451 (0.9543, -15.9664) -> (0.9543, -15.7175)
  line L1452 (0.9543, -15.7175) -> (1.1543, -15.7175)
  line L1453 (1.1543, -15.7175) -> (1.1543, -15.748)
  line L1454 (0.9543, -15.9964) -> (0.9543, -15.9664)
  line L1455 (1.1544, -14.722) -> (0.9544, -14.722)
  line L1456 (0.9544, -14.722) -> (0.9544, -14.4731)
  line L1457 (-0.7456, -14.7218) -> (0.7544, -14.7219)
  line L1458 (0.7544, -14.7219) -> (0.7543, -15.7175)
  line L1459 (0.7543, -15.7175) -> (-0.7457, -15.7174)
  line L1460 (-0.7457, -15.7174) -> (-0.7456, -14.7218)
  line L1461 (0.7544, -14.7219) -> (0.6938, -14.8147)
  line L1462 (-0.7456, -14.7218) -> (-0.6851, -14.8146)
  line L1463 (-0.7457, -15.7174) -> (-0.6885, -15.691)
  line L1464 (0.7543, -15.7175) -> (0.6971, -15.6911)
  line L1465 (3.62, -17.1773) -> (3.8191, -17.1584)